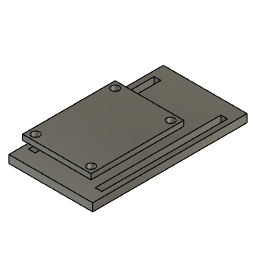
Case+Tarjeta+2+-+Tapa+headers (Autodesk Fusion 360 design; units mm, degrees)
Autodesk Fusion 360 part; units mm, degrees
sketch "Boceto1" plane through (0, 0, 0) normal (0, 0, 1) x (1, 0, 0)
  line L0 (0, 0) -> (30, 0)
  line L1 (30, 0) -> (30, 57)
  line L2 (30, 57) -> (0, 57)
  line L3 (0, 57) -> (0, 0)
  dimension "d1" = 57
  dimension "d2" = 30
  constraint horizontal L0
  constraint vertical L1
  constraint horizontal L2
  constraint vertical L3
  constraint coincident L0.start L3.end
  measures "d1" distance of L0.end L1.end
  measures "d2" distance of L0.start L0.end
extrude "Extruir1" add sketch "Boceto1" along normal blind 3
sketch "Boceto2" plane through (0, 0, 3) normal (0, 0, 1) x (-1, 0, 0)
  line L0 (0, -57) -> (0, 0)
  line L1 (0, 0) -> (-30, 0)
  line L2 (-30, 0) -> (-30, -57)
  line L3 (-30, -57) -> (0, -57)
  line L4 (-0.98, -52.5) -> (-3.52, -52.5)
  line L5 (-3.52, -52.5) -> (-3.52, -4.5)
  line L6 (-3.52, -4.5) -> (-0.98, -4.5)
  line L7 (-0.98, -4.5) -> (-0.98, -52.5)
  line L8 (-15, -57) -> (-15, 0) construction
  line L9 (-26.48, -52.5) -> (-26.48, -4.5)
  line L10 (-29.02, -4.5) -> (-29.02, -52.5)
  line L11 (-29.02, -52.5) -> (-26.48, -52.5)
  line L12 (-26.48, -4.5) -> (-29.02, -4.5)
  point P0 (-0.98, -28.5)
  point P1 (0, -28.5)
  point P2 (-2.25, -52.5)
  point P3 (-27.75, -52.5)
  dimension "d5" = 2.54
  dimension "d6" = 48
  dimension "d7" = 25.5
  constraint horizontal L4
  constraint vertical L5
  constraint horizontal L6
  constraint vertical L7
  constraint midpoint L7 P0
  constraint midpoint L0 P1
  constraint horizontal P0 P1
  constraint midpoint L3 L8.start
  constraint midpoint L1 L8.end
  constraint symmetric L4.start L8 L10.end
  constraint symmetric L4.end L8 L9.start
  constraint symmetric L5.end L8 L9.end
  constraint symmetric L6.end L8 L10.start
  constraint midpoint L4 P2
  constraint midpoint L11 P3
  measures "d5" distance of L4.start L4.end
  measures "d6" distance of L4.start L6.end
  measures "d7" distance of P2 P3
extrude "Extruir2" cut sketch "Boceto2" against normal through all contours L4 L5 L6 L7 | L9 L10 L11 L12
sketch "Boceto3" plane through (0, 0, 3) normal (0, 0, 1) x (-1, 0, 0)
  line L0 (-0.98, -4.5) -> (-0.98, -52.5)
  line L1 (-0.98, -52.5) -> (-3.52, -52.5)
  line L2 (-3.52, -52.5) -> (-3.52, -4.5)
  line L3 (-3.52, -4.5) -> (-0.98, -4.5)
  line L4 (-26.48, -4.5) -> (-26.48, -52.5)
  line L5 (-26.48, -52.5) -> (-29.02, -52.5)
  line L6 (-29.02, -52.5) -> (-29.02, -4.5)
  line L7 (-29.02, -4.5) -> (-26.48, -4.5)
  line L8 (0, -57) -> (0, 0)
  line L9 (0, 0) -> (-30, 0)
  line L10 (-30, 0) -> (-30, -57)
  line L11 (-30, -57) -> (0, -57)
  line L12 (1, -58) -> (1, 1)
  line L13 (1, 1) -> (-31, 1)
  line L14 (-31, 1) -> (-31, -58)
  line L15 (-31, -58) -> (1, -58)
  dimension "d9" = 1
extrude "Extruir3" add sketch "Boceto3" against normal up to surface (3 mm away) contours L12 L13 L14 L15
sketch "Boceto4" plane through (0, 0, 3) normal (0, 0, 1) x (-1, 0, 0)
  line L0 (-31, -58) -> (1, -58)
  line L1 (1, -58) -> (1, 1)
  line L2 (1, 1) -> (-31, 1)
  line L3 (-31, 1) -> (-31, -58)
  line L4 (-0.98, -4.5) -> (-0.98, -52.5)
  line L5 (-0.98, -52.5) -> (-3.52, -52.5)
  line L6 (-3.52, -52.5) -> (-3.52, -4.5)
  line L7 (-3.52, -4.5) -> (-0.98, -4.5)
  line L8 (-26.48, -4.5) -> (-26.48, -52.5)
  line L9 (-26.48, -52.5) -> (-29.02, -52.5)
  line L10 (-29.02, -52.5) -> (-29.02, -4.5)
  line L11 (-29.02, -4.5) -> (-26.48, -4.5)
  line L12 (-22, -9) -> (-8, -9)
  line L13 (-8, -9) -> (-8, -29)
  line L14 (-8, -29) -> (-22, -29)
  line L15 (-22, -29) -> (-22, -9)
  point P0 (-15, -9)
  point P1 (-15, 1)
  dimension "d12" = 10
  dimension "d13" = 20
  dimension "d14" = 14
  constraint horizontal L12
  constraint vertical L13
  constraint horizontal L14
  constraint vertical L15
  constraint midpoint L12 P0
  constraint midpoint L2 P1
  constraint vertical P0 P1
  measures "d12" distance of L2 L12
  measures "d13" distance of L12.end L13.end
  measures "d14" distance of L13.end L14.end
extrude "Extruir4" add sketch "Boceto4" along normal blind 5 contours L12 L13 L14 L15
sketch "Boceto5" plane through (0, 0, 8) normal (0, 0, 1) x (-1, 0, 0)
  line L0 (-22, -29) -> (-8, -29)
  line L1 (-8, -29) -> (-8, -9)
  line L2 (-8, -9) -> (-22, -9)
  line L3 (-22, -9) -> (-22, -29)
  line L4 (-28.1, -1.3) -> (-1.9, -1.3)
  line L5 (-1.9, -1.3) -> (-1.9, -36.7)
  line L6 (-1.9, -36.7) -> (-28.1, -36.7)
  line L7 (-28.1, -36.7) -> (-28.1, -1.3)
  line L8 (-25.6, -3.8) -> (-4.4, -3.8)
  line L9 (-4.4, -3.8) -> (-4.4, -34.2)
  line L10 (-4.4, -34.2) -> (-25.6, -34.2)
  line L11 (-25.6, -34.2) -> (-25.6, -3.8)
  circle A0 centre (-25.6, -3.8) radius 1.5
  circle A1 centre (-4.4, -3.8) radius 1.5
  circle A2 centre (-25.6, -34.2) radius 1.5
  circle A3 centre (-4.4, -34.2) radius 1.5
  point P0 (-15, -1.3)
  point P1 (-15, -9)
  point P2 (-1.9, -19)
  point P3 (-8, -19)
  point P4 (-15, -3.8)
  point P5 (-4.4, -19)
  dimension "d17" = 26.2
  dimension "d18" = 35.4
  dimension "d21" = 3
  dimension "d22" = 21.2
  dimension "d23" = 30.4
  constraint horizontal L4
  constraint vertical L5
  constraint horizontal L6
  constraint vertical L7
  constraint midpoint L4 P0
  constraint midpoint L2 P1
  constraint vertical P0 P1
  constraint midpoint L5 P2
  constraint midpoint L1 P3
  constraint horizontal P2 P3
  constraint horizontal L8
  constraint vertical L9
  constraint horizontal L10
  constraint vertical L11
  constraint midpoint L8 P4
  constraint vertical P0 P4
  constraint midpoint L9 P5
  constraint horizontal P2 P5
  constraint coincident L8.start L11.end
  constraint coincident L8.end L9.start
  constraint coincident L10.end L11.start
  constraint coincident L9.end L10.start
  constraint equal A0 A2
  constraint equal A1 A2
  constraint equal A1 A3
  measures "d17" distance of L5.end L6.end
  measures "d18" distance of L4.end L5.end
  measures "d21" diameter of A0
  measures "d22" distance of L8.start L8.end
  measures "d23" distance of L8.end L9.end
extrude "Extruir5" add sketch "Boceto5" along normal blind 2 contours L0 L1 L2 L3 | L4 L5 L6 L7 | L8 L9 L10 L11 A0 A1 A2 A3
